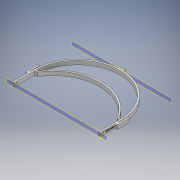
# Autodesk Inventor part: CARETA
Saved by Autodesk Inventor 2018 (Build 220112000, 112)
## iProperties
Created: 2020-04-02
Part Number: CARETA
Material: Generic
Document SubType Name: Modeling
Designer: paladín
Density: 1 g/cm^3
Appearance: Default
Author: paladín
Autodesk Inventor part; units mm, degrees
note: some values were not read from the file. Chosen so that the rebuilt part matches the saved one: direction of "Emboss1".
ref_plane "YZ Plane" through (0, 0, 0) normal (1, 0, 0) x (0, 1, 0)
ref_plane "XY Plane" through (0, 0, 0) normal (0, 0, 1) x (1, 0, 0)
sketch "Sketch2" plane through (0, 0, 0) normal (0, 0, 1) x (1, 0, 0)
  line L0 (0, 0) -> (200, 0) construction
  line L1 (200, 0) -> (200, 200) construction
  line L2 (200, 200) -> (0, 200) construction
  line L3 (0, 200) -> (0, 0) construction
  line L4 (6.0805, 0) -> (6.0805, 45)
  line L5 (182.0805, 45) -> (182.0805, 0)
  arc A0 (182.0805, 45) -> (6.0805, 45) centre (94.0805, 41.965) ccw
  line L6 (9.0805, 44.3568) -> (14.0805, 44.3568)
  line L7 (14.0805, 41.3424) -> (9.0805, 41.3424)
  line L8 (179.0805, 44.3568) -> (174.0805, 44.3568)
  line L9 (174.0805, 41.3568) -> (179.0805, 41.3568)
  arc A1 (175.13, 44.3568) -> (13.3559, 44.3568) centre (94.243, -6.137) ccw
  arc A2 (174.0805, 41.3568) -> (14.0805, 41.3424) centre (94.0849, -7.5382) ccw
  line L10 (6.0805, 0) -> (9.0805, 0)
  line L11 (182.0805, 0) -> (179.0805, 0)
  arc A3 (179.0805, 44.3568) -> (9.0805, 44.3568) centre (94.0805, 41.9844) ccw
  line L12 (9.0805, 41.3424) -> (9.0805, 0)
  line L13 (9.0805, 0) -> (6.0805, 0)
  line L14 (179.0805, 41.3568) -> (179.0805, 0)
  line L15 (179.0805, 0) -> (182.0805, 0)
  dimension "d33" = 200
  dimension "d34" = 200
  dimension "d35" = 45
  dimension "d39" = 45
  dimension "d44" = 5
  dimension "d45" = 3.0144
  dimension "d46" = 3
  dimension "d47" = 5
  dimension "d51" = 95.3537
  dimension "d52" = 93.7551
  dimension "d54" = 88.0523
  dimension "d55" = 17.9195
  dimension "d58" = 24.87
  dimension "d59" = 105.757
  dimension "d61" = 85.0331
  dimension "d62" = 41.3568
  dimension "d63" = 44.3568
  dimension "d64" = 44.3568
  dimension "d65" = 41.3424
  dimension "d68" = 105.9151
  dimension "d69" = 105.9195
  dimension "d70" = 3
  dimension "d71" = 20.9195
  dimension "d72" = 20.9195
  constraints: 32 end point, 8 point on circle, 6 point on line, 4 centre point, 4 horizontal, 4 parallel, 4 perpendicular, 3 vertical, 1 collinear
  measures "d33" distance of L1.end L2.end
  measures "d34" distance of L0.end L1.end
  measures "d35" distance of L4.start L4.end
  measures "d39" distance of L5.start L5.end
  measures "d44" distance of L7.start L7.end
  measures "d45" distance of L6.end L7.start
  measures "d46" distance of L8.end L9.start
  measures "d47" distance of L9.start L9.end
  measures "d51" radius of A1
  measures "d52" radius of A2
  measures "d54" radius of A0
  measures "d55" distance between parallel lines of L5 L1
  measures "d58" distance from line of A1.start L1
  measures "d59" distance from line of A1.centre L1
  measures "d61" radius of A3
  measures "d62" distance between parallel lines of L9 L11
  measures "d63" distance between parallel lines of L8 L11
  measures "d64" distance between parallel lines of L6 L11
  measures "d65" distance between parallel lines of L7 L11
  measures "d68" distance from line of A2.centre L1
  measures "d69" distance from line of A3.centre L1
  measures "d70" distance between parallel lines of L12 L4
  measures "d71" distance between parallel lines of L14 L1
  measures "d72" distance from line of L8.start L1
extrude "Extrusion1" add sketch "Sketch2" along normal blind 8
sketch "Sketch3" plane through (182.0805, 0, 0) normal (1, 0, 0) x (0, 0, -1)
  line L0 (-4, 14.6704) -> (-4, 2.726) construction
  line L1 (0, 0) -> (0, 45) projected
  line L2 (-6.1031, 18.2907) -> (-6.1031, 43.7602) construction
  line L3 (-6.1031, 43.7602) -> (-1.9659, 43.7602) construction
  line L4 (-1.9659, 43.7602) -> (-1.9659, 18.2907) construction
  line L5 (-1.9659, 18.2907) -> (-6.1031, 18.2907) construction
  line L6 (-6, 6.5211) -> (-2, 6.5211) construction
  line L7 (-4.3259, 4.847) -> (-3.6741, 4.847)
  line L8 (-3.6741, 8.1952) -> (-4.3259, 8.1952)
  arc A0 (-4.3259, 8.1952) -> (-4.3259, 4.847) centre (-4.3259, 6.5211) ccw
  arc A1 (-3.6741, 4.847) -> (-3.6741, 8.1952) centre (-3.6741, 6.5211) ccw
  line L9 (-8, 0) -> (-8, 45) projected
  point P0 (-4, 8.6982)
  point P1 (-4, 6.5211)
  dimension "d79" = 2
  dimension "d80" = 4
  dimension "d81" = 1.6741
  dimension "d82" = 4
  dimension "d83" = 1.9659
  dimension "d84" = 6.1031
  dimension "d85" = 37.2391
  dimension "d86" = 11.7696
  dimension "d87" = 36.8048
  dimension "d88" = 6.4752
  dimension "d89" = 0.503
  constraints: 12 end point, 6 point on circle, 4 tangent, 2 centre point, 2 midpoint, 2 parallel, 2 point on line, 1 horizontal, 1 vertical, 2 other
  measures "d79" distance edge to line of A0 L9
  measures "d80" distance of L6.start L6.end
  measures "d81" radius of A1
  measures "d82" distance between parallel lines of L1 L0
  measures "d83" distance between parallel lines of L4 L1
  measures "d84" distance between parallel lines of L2 L1
  measures "d85" distance between parallel lines of L3 L6
  measures "d86" distance between parallel lines of L5 L6
  measures "d87" distance from line of L1.end L8
  measures "d88" distance from line of L0.start L8
  measures "d89" distance from line of point (-4, 8.698) L8
extrude "Extrusion2" add sketch "Sketch3" against normal blind 3
sketch "Sketch4" plane through (182.0805, 0, 0) normal (1, 0, 0) x (0, 0, -1)
  line L0 (-6, 5.2531) -> (-2, 5.2531) construction
  line L1 (-4.5529, 3.806) -> (-3.4471, 3.806)
  line L2 (-3.4471, 6.7002) -> (-4.5529, 6.7002)
  arc A0 (-4.5529, 6.7002) -> (-4.5529, 3.806) centre (-4.5529, 5.2531) ccw
  arc A1 (-3.4471, 3.806) -> (-3.4471, 6.7002) centre (-3.4471, 5.2531) ccw
  line L3 (-8, 0) -> (-8, 45) projected
  point P0 (0, 0)
  point P1 (-4, 5.2531)
  dimension "d92" = 2
  dimension "d93" = 4
  dimension "d94" = 1.4471
  dimension "d95" = 6.7002
  constraints: 8 end point, 6 point on circle, 4 tangent, 2 centre point, 2 point on line, 1 horizontal, 1 midpoint, 1 parallel
  measures "d92" distance edge to line of A0 L3
  measures "d93" distance of L0.start L0.end
  measures "d94" radius of A1
  measures "d95" distance from line of point (0, 0) L2
extrude "Extrusion3" cut sketch "Sketch4" against normal blind 3
sketch "Sketch5" plane through (182.0805, 0, 0) normal (1, 0, 0) x (0, 0, -1)
  line L0 (-5.8835, 9.554) -> (-5.8835, 28.6561) construction
  line L1 (-5.8835, 28.6561) -> (-2.7806, 28.6561) construction
  line L2 (-2.7806, 28.6561) -> (-2.7806, 9.554) construction
  line L3 (-2.7806, 9.554) -> (-5.8835, 9.554) construction
  line L4 (-2.831, 9.8856) -> (-5.831, 9.8856)
  line L5 (-5.831, 9.8856) -> (-5.831, 12.0578)
  line L6 (-5.831, 12.0578) -> (-5.4765, 12.0578)
  line L7 (-5.4765, 12.0578) -> (-5.4765, 10.2834)
  line L8 (-5.4765, 10.2834) -> (-4.5596, 10.2834)
  line L9 (-4.5596, 10.2834) -> (-4.5596, 11.9458)
  line L10 (-4.5596, 11.9458) -> (-4.2052, 11.9458)
  line L11 (-4.2052, 11.9458) -> (-4.2052, 10.2834)
  line L12 (-4.2052, 10.2834) -> (-3.1854, 10.2834)
  line L13 (-3.1854, 10.2834) -> (-3.1854, 12.1264)
  line L14 (-3.1854, 12.1264) -> (-2.831, 12.1264)
  line L15 (-2.831, 12.1264) -> (-2.831, 9.8856)
  line L16 (-2.831, 12.6569) -> (-5.831, 12.6569)
  line L17 (-5.831, 12.6569) -> (-5.831, 13.7819)
  spline S0 degree 2 poles (-5.831, 13.7819) (-5.831, 14.1249) (-5.648, 14.5411) (-5.2707, 14.7766) (-5.0627, 14.7766) knots 0 0 0 1 2 3 3 3
  spline S1 degree 2 poles (-5.0627, 14.7766) (-4.8706, 14.7766) (-4.5322, 14.5685) (-4.427, 14.3558) knots 0 0 0 1 2 2 2
  spline S2 degree 2 poles (-4.427, 14.3558) (-4.347, 14.6302) (-3.9628, 14.9229) (-3.6999, 14.9229) knots 0 0 0 1 2 2 2
  spline S3 degree 2 poles (-3.6999, 14.9229) (-3.4895, 14.9229) (-3.1282, 14.7446) (-2.9316, 14.4839) (-2.831, 14.0883) (-2.831, 13.8002) knots 0 0 0 1 2 3 4 4 4
  line L18 (-2.831, 13.8002) -> (-2.831, 12.6569)
  line L19 (-3.1854, 13.0548) -> (-3.1854, 13.8025)
  spline S4 degree 2 poles (-3.1854, 13.8025) (-3.1854, 13.9946) (-3.1991, 14.0723) knots 0 0 0 1 1 1
  spline S5 degree 2 poles (-3.1991, 14.0723) (-3.2242, 14.2095) (-3.3386, 14.3947) (-3.5581, 14.5136) (-3.7021, 14.5136) knots 0 0 0 1 2 3 3 3
  spline S6 degree 2 poles (-3.7021, 14.5136) (-3.8691, 14.5136) (-4.116, 14.3375) (-4.2166, 14.0334) (-4.2166, 13.7476) knots 0 0 0 1 2 3 3 3
  line L20 (-4.2166, 13.7476) -> (-4.2166, 13.0548)
  line L21 (-4.2166, 13.0548) -> (-3.1854, 13.0548)
  line L22 (-4.571, 13.0548) -> (-4.571, 13.7019)
  spline S7 degree 2 poles (-4.571, 13.7019) (-4.571, 13.9671) (-4.6053, 14.0815) knots 0 0 0 1 1 1
  spline S8 degree 2 poles (-4.6053, 14.0815) (-4.6511, 14.2324) (-4.8592, 14.3856) (-5.0169, 14.3856) knots 0 0 0 1 2 2 2
  spline S9 degree 2 poles (-5.0169, 14.3856) (-5.1656, 14.3856) (-5.3919, 14.2415) (-5.4765, 13.9763) (-5.4765, 13.6539) knots 0 0 0 1 2 3 3 3
  line L23 (-5.4765, 13.6539) -> (-5.4765, 13.0548)
  line L24 (-5.4765, 13.0548) -> (-4.571, 13.0548)
  line L25 (-2.831, 15.538) -> (-5.831, 15.538)
  line L26 (-5.831, 15.538) -> (-5.831, 15.9359)
  line L27 (-5.831, 15.9359) -> (-2.831, 15.9359)
  line L28 (-2.831, 15.9359) -> (-2.831, 15.538)
  spline S10 degree 2 poles (-4.2921, 16.5144) (-5.0398, 16.5144) (-5.8835, 17.317) (-5.8835, 17.9504) knots 0 0 0 1 2 2 2
  spline S11 degree 2 poles (-5.8835, 17.9504) (-5.8835, 18.3665) (-5.4857, 19.0342) (-4.7768, 19.384) (-4.3264, 19.384) knots 0 0 0 1 2 3 3 3
  spline S12 degree 2 poles (-4.3264, 19.384) (-3.8713, 19.384) (-3.1511, 19.0159) (-2.7806, 18.3391) (-2.7806, 17.9504) knots 0 0 0 1 2 3 3 3
  spline S13 degree 2 poles (-2.7806, 17.9504) (-2.7806, 17.525) (-3.1899, 16.8574) (-3.8965, 16.5144) (-4.2921, 16.5144) knots 0 0 0 1 2 3 3 3
  spline S14 degree 2 poles (-4.2875, 16.9237) (-3.7456, 16.9237) (-3.1213, 17.5068) (-3.1213, 17.9481) knots 0 0 0 1 2 2 2
  spline S15 degree 2 poles (-3.1213, 17.9481) (-3.1213, 18.3962) (-3.7502, 18.9747) (-4.331, 18.9747) knots 0 0 0 1 2 2 2
  spline S16 degree 2 poles (-4.331, 18.9747) (-4.6968, 18.9747) (-5.2433, 18.7278) (-5.5428, 18.2499) (-5.5428, 17.9526) knots 0 0 0 1 2 3 3 3
  spline S17 degree 2 poles (-5.5428, 17.9526) (-5.5428, 17.5319) (-4.9643, 16.9237) (-4.2875, 16.9237) knots 0 0 0 1 2 2 2
  line L29 (-2.831, 19.8825) -> (-5.831, 19.8825)
  line L30 (-5.831, 19.8825) -> (-5.831, 20.4793)
  line L31 (-5.831, 20.4793) -> (-3.7067, 21.1904)
  spline S18 degree 2 poles (-3.7067, 21.1904) (-3.4095, 21.2888) (-3.2631, 21.3345) knots 0 0 0 1 1 1
  spline S19 degree 2 poles (-3.2631, 21.3345) (-3.4255, 21.3848) (-3.7433, 21.4946) knots 0 0 0 1 1 1
  line L32 (-3.7433, 21.4946) -> (-5.831, 22.2148)
  line L33 (-5.831, 22.2148) -> (-5.831, 22.7476)
  line L34 (-5.831, 22.7476) -> (-2.831, 22.7476)
  line L35 (-2.831, 22.7476) -> (-2.831, 22.3657)
  line L36 (-2.831, 22.3657) -> (-5.3416, 22.3657)
  line L37 (-5.3416, 22.3657) -> (-2.831, 21.49)
  line L38 (-2.831, 21.49) -> (-2.831, 21.1333)
  line L39 (-2.831, 21.1333) -> (-5.3851, 20.2644)
  line L40 (-5.3851, 20.2644) -> (-2.831, 20.2644)
  line L41 (-2.831, 20.2644) -> (-2.831, 19.8825)
  line L42 (-2.831, 23.3947) -> (-5.831, 23.3947)
  line L43 (-5.831, 23.3947) -> (-5.831, 25.567)
  line L44 (-5.831, 25.567) -> (-5.4765, 25.567)
  line L45 (-5.4765, 25.567) -> (-5.4765, 23.7926)
  line L46 (-5.4765, 23.7926) -> (-4.5596, 23.7926)
  line L47 (-4.5596, 23.7926) -> (-4.5596, 25.4549)
  line L48 (-4.5596, 25.4549) -> (-4.2052, 25.4549)
  line L49 (-4.2052, 25.4549) -> (-4.2052, 23.7926)
  line L50 (-4.2052, 23.7926) -> (-3.1854, 23.7926)
  line L51 (-3.1854, 23.7926) -> (-3.1854, 25.6356)
  line L52 (-3.1854, 25.6356) -> (-2.831, 25.6356)
  line L53 (-2.831, 25.6356) -> (-2.831, 23.3947)
  line L54 (-2.831, 25.8779) -> (-4.3858, 27.0372)
  line L55 (-4.3858, 27.0372) -> (-5.831, 26.0151)
  line L56 (-5.831, 26.0151) -> (-5.831, 26.4862)
  line L57 (-5.831, 26.4862) -> (-5.0627, 27.035)
  spline S20 degree 2 poles (-5.0627, 27.035) (-4.8249, 27.2065) (-4.6945, 27.275) knots 0 0 0 1 1 1
  spline S21 degree 2 poles (-4.6945, 27.275) (-4.8546, 27.3757) (-5.0329, 27.5151) knots 0 0 0 1 1 1
  line L58 (-5.0329, 27.5151) -> (-5.831, 28.1142)
  line L59 (-5.831, 28.1142) -> (-5.831, 28.5464)
  line L60 (-5.831, 28.5464) -> (-4.4041, 27.506)
  line L61 (-4.4041, 27.506) -> (-2.831, 28.6287)
  line L62 (-2.831, 28.6287) -> (-2.831, 28.1417)
  line L63 (-2.831, 28.1417) -> (-3.9011, 27.3825)
  spline S22 degree 2 poles (-3.9011, 27.3825) (-3.9925, 27.3185) (-4.0863, 27.2568) knots 0 0 0 1 1 1
  spline S23 degree 2 poles (-4.0863, 27.2568) (-3.9331, 27.1584) (-3.8713, 27.115) knots 0 0 0 1 1 1
  line L64 (-3.8713, 27.115) -> (-2.831, 26.3558)
  line L65 (-2.831, 26.3558) -> (-2.831, 25.8779)
  point P0 (0, 0)
  constraints: 2 other
emboss "Emboss1" sketch "Sketch5" operation cut depth 1 direction (-1, 0, 0)
sketch "Sketch6" plane through (182.0805, 0, 0) normal (1, 0, 0) x (0, 0, -1)
  point P0 (0, 0)
sketch "Sketch7" plane through (6.0805, 0, 0) normal (-1, 0, 0) x (0, 0, 1)
  line L0 (6, 5.2915) -> (2, 5.2915) construction
  line L1 (4.5085, 6.7831) -> (3.4915, 6.7831)
  line L2 (3.4915, 3.8) -> (4.5085, 3.8)
  arc A0 (4.5085, 3.8) -> (4.5085, 6.7831) centre (4.5085, 5.2915) ccw
  arc A1 (3.4915, 6.7831) -> (3.4915, 3.8) centre (3.4915, 5.2915) ccw
  line L3 (0, 0) -> (8, 0) projected
  line L4 (0, 45) -> (0, 0) projected
  point P0 (4, 5.2915)
  dimension "d100" = 4
  dimension "d101" = 3.8
  dimension "d102" = 2
  dimension "d103" = 1.4915
  constraints: 8 end point, 6 point on circle, 4 tangent, 2 centre point, 2 point on line, 1 horizontal, 1 midpoint, 1 parallel
  measures "d100" distance of L0.start L0.end
  measures "d101" distance between parallel lines of L2 L3
  measures "d102" distance edge to line of A1 L4
  measures "d103" radius of A0
extrude "Extrusion4" cut sketch "Sketch7" against normal blind 3
sketch "Sketch8" plane through (6.0805, 0, 0) normal (-1, 0, 0) x (0, 0, 1)
  line L0 (0, 30) -> (8, 30)
  line L1 (8, 30) -> (8, 35)
  line L2 (8, 35) -> (0, 35)
  line L3 (0, 35) -> (0, 30)
  line L4 (0, 45) -> (8, 45) projected
  point P0 (0, 0)
  dimension "d106" = 5
  dimension "d107" = 8
  dimension "d108" = 10
  dimension "d109" = 0
  constraints: 8 end point, 2 parallel, 1 horizontal, 1 perpendicular
  measures "d106" distance between parallel lines of L2 L0
  measures "d107" distance between parallel lines of L1 L3
  measures "d108" distance between parallel lines of L4 L2
  measures "d109" distance from line of L4.end L1
extrude "Extrusion5" add sketch "Sketch8" along normal blind 1
sketch "Sketch9" plane through (5.0805, 0, 0) normal (-1, 0, 0) x (0, 0, 1)
  point P0 (0, 0)
sketch "Sketch10" plane through (5.0805, 0, 0) normal (-1, 0, 0) x (0, 0, 1)
  line L0 (8, 30) -> (0, 30) projected
  line L1 (0, 30) -> (8, 30)
  line L2 (8, 30) -> (8, 55)
  line L3 (8, 55) -> (0, 55)
  line L4 (0, 55) -> (0, 30)
  point P0 (0, 0)
  dimension "d112" = 25
  dimension "d113" = 8
  constraints: 8 end point, 2 parallel, 1 horizontal, 1 perpendicular
  measures "d112" distance between parallel lines of L3 L0
  measures "d113" distance between parallel lines of L2 L4
extrude "Extrusion6" add sketch "Sketch10" along normal blind 3
sketch "Sketch11" plane through (182.0805, 0, 0) normal (1, 0, 0) x (0, 0, -1)
  line L0 (-8, 0) -> (-8, 45) projected
  line L1 (-8, 30) -> (0, 30)
  line L2 (0, 30) -> (0, 35)
  line L3 (0, 35) -> (-8, 35)
  line L4 (-8, 35) -> (-8, 30)
  line L5 (0, 0) -> (-8, 0) projected
  dimension "d116" = 30
  dimension "d117" = 5
  dimension "d118" = 8
  constraints: 8 end point, 2 parallel, 1 horizontal, 1 perpendicular, 1 point on line
  measures "d116" distance between parallel lines of L1 L5
  measures "d117" distance between parallel lines of L3 L1
  measures "d118" distance between parallel lines of L0 L2
extrude "Extrusion7" add sketch "Sketch11" along normal blind 1
sketch "Sketch12" plane through (183.0805, 0, 0) normal (1, 0, 0) x (0, 0, -1)
  line L0 (-8, 30) -> (0, 30) projected
  line L1 (-8, 30) -> (0, 30)
  line L2 (0, 30) -> (0, 55)
  line L3 (0, 55) -> (-8, 55)
  line L4 (-8, 55) -> (-8, 30)
  point P0 (0, 0)
  dimension "d121" = 25
  dimension "d122" = 8
  constraints: 8 end point, 2 parallel, 1 horizontal, 1 perpendicular
  measures "d121" distance between parallel lines of L3 L0
  measures "d122" distance between parallel lines of L2 L4
extrude "Extrusion8" add sketch "Sketch12" along normal blind 3
ref_plane "Work Plane1" through (0, 130, 0) normal (0, 1, 0) x (-1, 0, 0)
sketch "Sketch13" plane through (0, 130, 0) normal (0, 1, 0) x (-1, 0, 0)
  line L0 (-2.0805, 8) -> (-2.0805, 0) projected
  line L1 (-174.0805, 8) -> (-14.0805, 8) projected
  line L2 (-90.726, 8) -> (-97.726, 8)
  line L3 (-97.726, 8) -> (-97.726, 5)
  line L4 (-97.726, 5) -> (-90.726, 5)
  line L5 (-90.726, 5) -> (-90.726, 8)
  point P0 (0, 0)
  dimension "d128" = 3
  dimension "d129" = 7
  dimension "d130" = 88.6455
  constraints: 8 end point, 2 parallel, 1 horizontal, 1 perpendicular, 1 point on line
  measures "d128" distance of L4.end L2.start
  measures "d129" distance of L3.end L4.end
  measures "d130" distance between parallel lines of L0 L5
extrude "Extrusion9" add sketch "Sketch13" along normal mid plane 2
sketch "Sketch14" plane through (0, 131, 0) normal (0, 1, 0) x (1, 0, 0)
  line L0 (91.2266, -7.9998) -> (98.1958, -7.9998)
  line L1 (98.1958, -7.9998) -> (98.1958, -0.7128)
  line L2 (98.1958, -0.7128) -> (91.2266, -0.7128)
  line L3 (91.2266, -0.7128) -> (91.2266, -7.9998)
  point P0 (0, 0)
  dimension "d133" = 6.9692
  dimension "d134" = 7.287
  dimension "d135" = 98.1958
  dimension "d136" = 0.7128
  constraints: 8 end point, 2 parallel, 1 horizontal, 1 perpendicular
  measures "d133" distance between parallel lines of L1 L3
  measures "d134" distance between parallel lines of L0 L2
  measures "d135" distance from line of point (0, 0) L1
  measures "d136" distance from line of point (0, 0) L2
extrude "Extrusion10" add sketch "Sketch14" along normal blind 3
body "Solid1"
